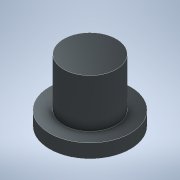
# Autodesk Inventor part: armscrew
Saved by Autodesk Inventor 2021 (Build 250183000, 183)
## iProperties
Created: 2021-07-07
Part Number: armscrew
Material: Iron, Gray
Document SubType Name: Modeling
Designer: KAVYA
Density: 7.15 g/cm^3
Appearance: Iron Gray
Author: KAVYA
Autodesk Inventor part; units mm, degrees
ref_plane "YZ Plane" through (0, 0, 0) normal (1, 0, 0) x (0, 1, 0)
ref_plane "XZ Plane" through (0, 0, 0) normal (0, 1, 0) x (-1, 0, 0)
ref_plane "XY Plane" through (0, 0, 0) normal (0, 0, 1) x (1, 0, 0)
sketch "Sketch1" plane through (0, 0, 0) normal (0, 1, 0) x (-1, 0, 0)
  circle A0 centre (0, 0) radius 2.921
  dimension "d0" = 5.842
  constraints: 1 centre point, 1 coincident
  measures "d0" diameter of A0
extrude "Extrusion1" add sketch "Sketch1" along normal blind 1
sketch "Sketch2" plane through (0, 1, 0) normal (0, 1, 0) x (1, 0, 0)
  circle A0 centre (0, 0) radius 1.905
  dimension "d3" = 3.81
  constraints: 1 centre point, 1 coincident
  measures "d3" diameter of A0
extrude "Extrusion2" add sketch "Sketch2" along normal blind 3.5
sketch "Sketch3" plane through (0, 0, 0) normal (0, -1, 0) x (1, 0, 0)
  line L0 (0, 1.905) -> (-1, 1.905)
  line L1 (-1, -1.905) -> (1, -1.905)
  line L2 (1, 1.905) -> (0, 1.905)
  line L3 (-1.905, 0) -> (-1.905, -1)
  line L4 (1.905, -1) -> (1.905, 1)
  line L5 (-1.905, 0) -> (-1.905, 1)
  line L6 (-1.905, 1) -> (-1, 1)
  line L7 (1, 1) -> (1.905, 1)
  line L8 (1, -1.905) -> (1, -1)
  line L9 (1, 1) -> (1, 1.905)
  line L10 (-1.905, -1) -> (-1, -1)
  line L11 (1, -1) -> (1.905, -1)
  line L12 (-1, 1.905) -> (-1, 1)
  line L13 (-1, -1) -> (-1, -1.905)
  point P0 (0, 0)
  dimension "d7" = 1
  dimension "d8" = 3.81
  dimension "d9" = 2
  dimension "d10" = 3.81
  dimension "d11" = 1
  dimension "d12" = 3.81
  dimension "d13" = 2
  dimension "d15" = 1
  constraints: 28 end point, 8 perpendicular, 4 parallel, 1 horizontal, 1 point on line, 1 vertical
  measures "d7" distance of L0.start L0.end
  measures "d8" distance of L0.end L1.start
  measures "d9" distance of L1.start L1.end
  measures "d10" distance of L1.end L2.start
  measures "d11" distance of L3.start L3.end
  measures "d12" distance of L3.end L4.start
  measures "d13" distance of L4.start L4.end
  measures "d15" distance of L3.start L5.end
extrude "Extrusion3" cut sketch "Sketch3" against normal blind 0.5
body "Solid1"
